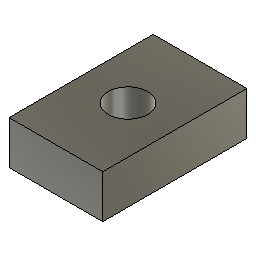
Inner Cover Mounts (Autodesk Fusion 360 design; units mm, degrees)
Autodesk Fusion 360 part; units mm, degrees
sketch "Sketch1" plane through (0, 0, 0) normal (0, 0, 1) x (1, 0, 0)
  line L0 (6.5, -10) -> (-6.5, -10)
  line L1 (-6.5, -10) -> (-6.5, 10)
  line L2 (-6.5, 10) -> (6.5, 10)
  line L3 (6.5, 10) -> (6.5, -10)
  line L4 (6.5, -10) -> (-6.5, 10) construction
  line L5 (-6.5, -10) -> (6.5, 10) construction
  circle A0 centre (0, 0) radius 2.75
  dimension "d1" = 13
  dimension "d2" = 20
  dimension "d3" = 5.5
  constraint horizontal L0
  constraint perpendicular L0 L1
  constraint parallel L0 L2
  constraint parallel L1 L3
  constraint coincident L4 A0.centre
  constraint coincident L5 A0.centre
  constraint coincident A0.centre origin
  measures "d1" distance of L1.end L2.end
  measures "d2" distance of L0.end L1.end
  measures "d3" diameter of A0
extrude "Extrude1" add sketch "Sketch1" along normal blind 6
